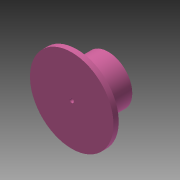
# Autodesk Inventor part: Part12
Saved by Autodesk Inventor 2015 (Build 190159000, 159)
## iProperties
Created: 2015-07-08
Part Number: Part12
Material: ABS Plastic
Document SubType Name: Modeling
Designer: eefred
Density: 1.06 g/cm^3
Appearance: Pink
Author: eefred
Autodesk Inventor part; units mm, degrees
ref_plane "YZ Plane" through (0, 0, 0) normal (1, 0, 0) x (0, 1, 0)
ref_plane "XZ Plane" through (0, 0, 0) normal (0, 1, 0) x (-1, 0, 0)
ref_plane "XY Plane" through (0, 0, 0) normal (0, 0, 1) x (1, 0, 0)
sketch "Sketch1" plane through (0, 0, 0) normal (1, 0, 0) x (0, 1, 0)
  line L0 (0, -2) -> (5, -2)
  line L1 (5, -2) -> (5, -19)
  line L2 (5, -19) -> (35, -19)
  line L3 (35, -19) -> (35, -23)
  line L4 (35, -23) -> (5, -23)
  line L5 (5, -23) -> (5, -40)
  line L6 (5, -40) -> (0, -40)
  line L7 (0, -40) -> (0, -2)
  line L8 (-7, 0) -> (42, 0) projected
  point P0 (0, 0)
  dimension "d0" = 35
  dimension "d1" = 2
  dimension "d2" = 5
  dimension "d3" = 19
  dimension "d4" = 23
  dimension "d5" = 40
  constraints: 16 end point, 6 perpendicular, 2 point on line, 1 horizontal, 1 vertical alignment
  measures "d0" distance between parallel lines of L7 L3
  measures "d1" distance from line of point (0, 0) L0
  measures "d2" distance of L5.end L6.end
  measures "d3" distance from line of point (0, 0) L2
  measures "d4" distance from line of point (0, 0) L4
  measures "d5" distance from line of point (0, 0) L6
revolve "Revolution1" add sketch "Sketch1" angle 360 about axis through (0, -10, 0) along (0, 1, 0)
body "Solid1"
